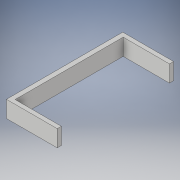
# Autodesk Inventor part: BoxHolders
Saved by Autodesk Inventor 2017 SP1 (Build 210196100, 196)
## iProperties
Created: 2018-01-06
Part Number: BoxHolders
Material: Generic
Document SubType Name: Modeling
Designer: 1452927
Density: 1 g/cm^3
Appearance: Default
Author: 1452927
Autodesk Inventor part; units mm, degrees
ref_plane "YZ Plane" through (0, 0, 0) normal (1, 0, 0) x (0, 1, 0)
ref_plane "XZ Plane" through (0, 0, 0) normal (0, 1, 0) x (-1, 0, 0)
ref_plane "XY Plane" through (0, 0, 0) normal (0, 0, 1) x (1, 0, 0)
sketch "Sketch1" plane through (0, 0, 0) normal (0, 1, 0) x (-1, 0, 0)
  line L0 (-35.3568, 82.55) -> (35.3568, 82.55)
  line L1 (35.3568, 82.55) -> (35.3568, -82.55)
  line L2 (35.3568, -82.55) -> (-35.3568, -82.55)
  line L3 (-35.3568, 82.55) -> (35.3568, -82.55) construction
  line L4 (35.3568, 82.55) -> (-35.3568, -82.55) construction
  line L5 (-35.3568, 88.9) -> (42.3418, 88.9)
  line L6 (42.3418, 88.9) -> (42.3418, -88.9)
  line L7 (42.3418, -88.9) -> (-35.3568, -88.9)
  line L8 (42.3418, 88.9) -> (-35.3568, -88.9) construction
  line L9 (42.3418, -88.9) -> (-35.3568, 88.9) construction
  line L10 (3.4925, 0) -> (42.3418, 0) construction
  line L11 (-35.3568, -88.9) -> (-35.3568, -82.55)
  line L12 (-35.3568, 82.55) -> (-35.3568, 88.9)
  point P0 (0, 0)
  point P1 (35.3568, 0)
  dimension "d1" = 165.1
  dimension "d2" = 177.8
  dimension "d3" = 77.6986
  dimension "d4" = 70.7136
  dimension "d5" = 70.7136
  constraints: 26 end point, 5 midpoint, 4 parallel, 2 horizontal, 2 perpendicular, 1 point on line
  measures "d1" distance of L0.end L1.end
  measures "d2" distance of L5.end L6.end
  measures "d3" distance of L5.start L5.end
  measures "d4" distance of L1.end L2.end
  measures "d5" distance of L0.start L0.end
extrude "Extrusion1" add sketch "Sketch1" along normal blind 25.4
body "Solid1"
